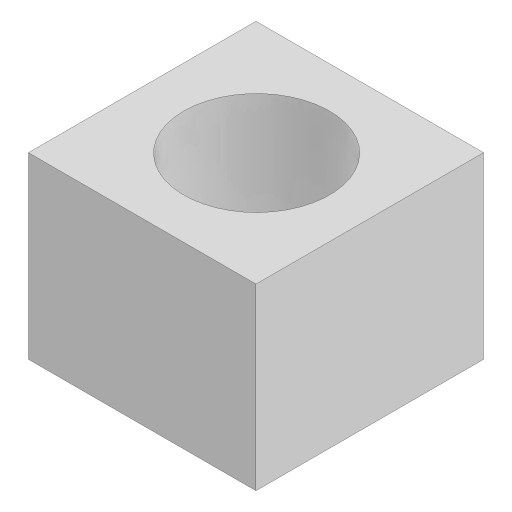
# Autodesk Inventor part: GDME Derivatizante
Saved by Autodesk Inventor 2024.3 (Build 283343000, 343)
## iProperties
Created: 2024-09-11
Part Number: GDME Derivatizante
Material: Genérico
Document SubType Name: Modeling
Designer: barof
Density: 1 g/cm^3
Appearance: Padrão
Author: barof
## iProperties of the stored document GDME Derivatizante_3DPrint.ipt
Created: 2024-09-11
Part Number: GDME Derivatizante_3DPrint
Material: Genérico
Document SubType Name: Modeling
Designer: barof
Density: 1 g/cm^3
Appearance: Padrão
Author: barof
Autodesk Inventor part; units mm, degrees
ref_plane "YZ Plane" through (0, 0, 0) normal (1, 0, 0) x (0, 1, 0)
ref_plane "XZ Plane" through (0, 0, 0) normal (0, 1, 0) x (-1, 0, 0)
ref_plane "XY Plane" through (0, 0, 0) normal (0, 0, 1) x (1, 0, 0)
sketch "Esboço1" plane through (0, 0, 0) normal (0, 1, 0) x (-1, 0, 0)
  line L0 (0, -67.2147) -> (17.8, -67.2147)
  line L1 (17.8, -67.2147) -> (17.8, -85.0147)
  line L2 (17.8, -85.0147) -> (0, -85.0147)
  line L3 (0, -85.0147) -> (0, -67.2147)
  circle A0 centre (8.85, -76.1147) radius 5.7
  point P0 (0, 0)
  dimension "d5" = 17.8
  dimension "d6" = 17.8
  dimension "d8" = 11.4
  constraints: 8 end point, 2 parallel, 1 centre point, 1 horizontal, 1 perpendicular
  measures "d5" distance of L1.end L2.end
  measures "d6" distance of L0.end L1.end
  measures "d8" diameter of A0
extrude "Extrusão1" add sketch "Esboço1" along normal blind 14
